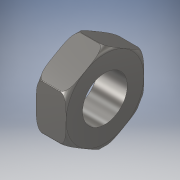
# Autodesk Inventor part: Nut
Saved by Autodesk Inventor 2017 (Build 210142000, 142)
## iProperties
Created: 2016-06-17
Part Number: Nut
Material: Steel, Carbon
Document SubType Name: Modeling
Designer: Dakota Marin
Density: 7.85 g/cm^3
Appearance: Semi-Polished
Author: Dakota Marin
Autodesk Inventor part; units mm, degrees
ref_plane "YZ Plane" through (0, 0, 0) normal (1, 0, 0) x (0, 1, 0)
ref_plane "XZ Plane" through (0, 0, 0) normal (0, 1, 0) x (-1, 0, 0)
ref_plane "XY Plane" through (0, 0, 0) normal (0, 0, 1) x (1, 0, 0)
sketch "Sketch4" plane through (0, 0, 0) normal (1, 0, 0) x (0, 1, 0)
  circle A0 centre (0, 0) radius 7.5
  circle A1 centre (0, 0) radius 15
  dimension "d12" = 15
  dimension "d13" = 30
  constraints: 2 centre point, 2 coincident
  measures "d12" diameter of A0
  measures "d13" diameter of A1
extrude "Extrusion3" add sketch "Sketch4" along normal blind 10
fillet "Fillet1" radius 2 2 edges at (10, -15, 0) (0, -15, 0)
sketch "Sketch6" plane through (10, 0, 0) normal (1, 0, 0) x (0, 0, -1)
  line L0 (-12.986, 7.6174) -> (0.1038, 15.0549)
  line L1 (0.1038, 15.0549) -> (13.0898, 7.4376)
  line L2 (13.0898, 7.4376) -> (12.986, -7.6174)
  line L3 (12.986, -7.6174) -> (-0.1038, -15.0549)
  line L4 (-0.1038, -15.0549) -> (-13.0898, -7.4376)
  line L5 (-13.0898, -7.4376) -> (-12.986, 7.6174)
  circle A0 centre (0, 0) radius 17.8514
  circle A1 centre (0, 0) radius 7.5945
  constraints: 12 end point, 3 coincident, 2 centre point, 13 other
extrude "Extrusion4" cut sketch "Sketch6" against normal blind 10 contours A0
body "Solid2"
